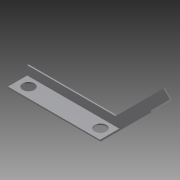
# Autodesk Inventor part: 8 ball bottom 1 by 2 L
Saved by Autodesk Inventor 2012 (Build 160160000, 160)
## iProperties
Created: 2013-10-10
Part Number: 8 ball bottom 1 by 2 L
Material: Default
Document SubType Name: Modeling
Designer: Bryce
Density: 1 g/cm^3
Author: Bryce
Autodesk Inventor part; units mm, degrees
ref_plane "YZ Plane" through (0, 0, 0) normal (1, 0, 0) x (0, 1, 0)
ref_plane "XZ Plane" through (0, 0, 0) normal (0, 1, 0) x (-1, 0, 0)
ref_plane "XY Plane" through (0, 0, 0) normal (0, 0, 1) x (1, 0, 0)
sketch "Sketch1" plane through (0, 0, 0) normal (0, 0, 1) x (1, 0, 0)
  line L0 (0, 0) -> (228.6, 0)
  line L1 (228.6, 0) -> (354.3236, 125.7236)
  line L2 (354.3236, 125.7236) -> (352.0785, 127.9686)
  line L3 (352.0785, 127.9686) -> (227.2849, 3.175)
  line L4 (0, 0) -> (0, 3.175)
  line L5 (0, 3.175) -> (227.2849, 3.175)
  line L6 (0, 3.175) -> (0, 25.4)
  line L7 (0, 25.4) -> (217.2198, 25.4)
  line L8 (352.0785, 127.9686) -> (336.3631, 143.6841)
  line L9 (336.3631, 143.6841) -> (218.6865, 26.0075)
  line L10 (217.2198, 25.4) -> (226.2228, 3.665)
  line L11 (218.6865, 26.0075) -> (227.6894, 4.2725)
  arc A0 (226.2228, 3.665) -> (227.6894, 4.2725) centre (226.9561, 3.9688) ccw
  line L12 (217.2198, 25.4) -> (218.079, 25.4) construction
  line L13 (218.6865, 26.0075) -> (218.079, 25.4) construction
  dimension "d4" = 3.175
  dimension "d6" = 3.175
  dimension "d8" = 25.4
  dimension "d9" = 25.4
  dimension "d10" = 45
  dimension "d11" = 228.6
  dimension "d12" = 177.8
  dimension "d13" = 1.5875
  constraints: 28 end point, 10 perpendicular, 4 tangent, 2 point on circle, 1 centre point, 1 equal length, 1 horizontal, 1 parallel
  measures "d4" distance of L0.start L4.end
  measures "d6" distance of L1.end L2.end
  measures "d8" distance between parallel lines of L9 L1
  measures "d9" distance between parallel lines of L7 L0
  measures "d10" angle of L0 L1
  measures "d11" distance of L0.start L0.end
  measures "d12" distance of L0.end L1.end
  measures "d13" distance between parallel lines of L10 L11
extrude "Extrusion1" add sketch "Sketch1" along normal blind 3.175 contours L6 L7 L10 A0 L5 | A0 L3 L5 | L3 A0 L11 L9 L8
extrude "Extrusion2" add sketch "Sketch1" along normal blind 50.8 contours L4 L5 L3 L2 L1 L0
sketch "Sketch2" plane through (0, 0, 0) normal (0, -1, 0) x (1, 0, 0)
  line L0 (0, 0) -> (0, 50.8) projected
  line L1 (0, 0) -> (228.6, 0) projected
  line L2 (228.6, 0) -> (228.6, 50.8) projected
  circle A0 centre (25.4, 25.4) radius 14.2875
  circle A1 centre (203.2, 25.4) radius 14.2875
  dimension "d18" = 28.575
  dimension "d19" = 25.4
  dimension "d20" = 25.4
  dimension "d21" = 25.4
  constraints: 2 centre point, 1 equal radius, 1 horizontal alignment
  measures "d18" diameter of A0
  measures "d19" distance from line of L0 A0.centre
  measures "d20" distance from line of L1 A0.centre
  measures "d21" distance from line of L2 A1.centre
extrude "Extrusion3" cut sketch "Sketch2" against normal through all
equation "\"d4\" = d6"
body "Solid1"
